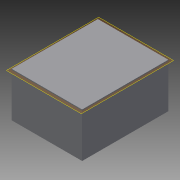
# Autodesk Inventor part: Deckel
Saved by Autodesk Inventor 2014 (Build 180170000, 170)
## iProperties
Created: 2016-09-06
Part Number: Deckel
Material: Generisch
Document SubType Name: Modeling
Designer: cem
Density: 1 g/cm^3
Appearance: Vorgabe
Author: cem
Autodesk Inventor part; units mm, degrees
ref_plane "YZ Plane" through (0, 0, 0) normal (1, 0, 0) x (0, 1, 0)
ref_plane "Arbeitsebene1" through (0, 0, 0.5) normal (0, 0, 1) x (1, 0, 0)
sketch "Skizze1" plane through (0, 0, 0.5) normal (0, 0, 1) x (1, 0, 0)
  line L0 (-33.9, -46.4) -> (-33.9, 46.4) projected
  line L1 (-33.9, 46.4) -> (33.9, 46.4) projected
  line L2 (33.9, 46.4) -> (33.9, -46.4) projected
  line L3 (33.9, -46.4) -> (-33.9, -46.4) projected
  line L4 (35, 47.5) -> (-35, 47.5) projected
  line L5 (-35, 47.5) -> (-35, -47.5) projected
  line L6 (-35, -47.5) -> (35, -47.5) projected
  line L7 (35, -47.5) -> (35, 47.5) projected
  line L8 (-36.1, 48.6) -> (36.1, 48.6)
  line L9 (36.1, 48.6) -> (36.1, -48.6)
  line L10 (36.1, -48.6) -> (-36.1, -48.6)
  line L11 (-36.1, -48.6) -> (-36.1, 48.6)
  point P0 (0, 0)
  dimension "d0" = 1.1
  constraints: 8 end point, 3 other
  measures "d0" distance between parallel lines of L8 L4
extrude "Extrusion1" add sketch "Skizze1" along normal blind 1 contours L0 L1 L2 L3 | L7 L6 L5 L4 | L8 L9 L10 L11
sketch "Skizze2" plane through (0, 0, 0.5) normal (0, 0, -1) x (-1, 0, 0)
  line L0 (36.1, 48.6) -> (-36.1, 48.6) projected
  line L1 (-36.1, 48.6) -> (-36.1, -48.6) projected
  line L2 (-36.1, -48.6) -> (36.1, -48.6) projected
  line L3 (36.1, -48.6) -> (36.1, 48.6) projected
  line L4 (-35.1, 47.6) -> (35.1, 47.6)
  line L5 (35.1, 47.6) -> (35.1, -47.6)
  line L6 (35.1, -47.6) -> (-35.1, -47.6)
  line L7 (-35.1, -47.6) -> (-35.1, 47.6)
  point P0 (0, 0)
  dimension "d3" = 1
  constraints: 8 end point, 3 other
  measures "d3" distance between parallel lines of L7 L1
ref_plane "Arbeitsebene2" through (-34.54, -42.79, -40) normal (0, 0, 1) x (1, 0, 0)
ref_plane "Arbeitsebene3" through (-32.5, -40, -41) normal (0, 0, -1) x (0, 1, 0)
extrude "Extrusion2" add sketch "Skizze2" along normal up to surface (41.5 mm away)
sketch "Skizze3" plane through (-36.1, -48.6, 1.5) normal (0, -1, 0) x (1, 0, 0)
  line L0 (0, -42.5) -> (72.2, -42.5) projected
  line L1 (33.6, -45.4928) -> (33.6, 6) construction
  circle A0 centre (33.6, -42.5) radius 10
  point P0 (36.1, -1.5)
  dimension "d6" = 20
  constraints: 2 end point, 2 point on line, 1 centre point, 1 perpendicular
  measures "d6" diameter of A0
extrude "Extrusion3" cut sketch "Skizze3" against normal up to surface (97.2 mm away)
